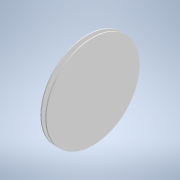
# Autodesk Inventor part: Base Plate
Saved by Autodesk Inventor 2021 (Build 250183000, 183)
## iProperties
Created: 2021-05-31
Part Number: Base Plate
Material: Generic
Document SubType Name: Modeling
Designer: techv
Density: 1 g/cm^3
Appearance: Default
Author: techv
Autodesk Inventor part; units mm, degrees
ref_plane "YZ Plane" through (0, 0, 0) normal (1, 0, 0) x (0, 1, 0)
ref_plane "XZ Plane" through (0, 0, 0) normal (0, 1, 0) x (-1, 0, 0)
ref_plane "XY Plane" through (0, 0, 0) normal (0, 0, 1) x (1, 0, 0)
sketch "Sketch1" plane through (0, 0, 0) normal (1, 0, 0) x (0, 1, 0)
  circle A0 centre (0, 0) radius 125
  dimension "d0" = 250
  constraints: 1 centre point, 1 coincident
  measures "d0" diameter of A0
extrude "Extrusion1" add sketch "Sketch1" along normal blind 3
sketch "Sketch2" plane through (3, 0, 0) normal (1, 0, 0) x (0, 0, -1)
  circle A0 centre (0, 0) radius 15
  line L0 (0, 0) -> (0, 70) construction
  circle A1 centre (0, 70) radius 7.5
  circle A2 centre (-49.4975, 49.4975) radius 7.5
  circle A3 centre (-70, 0) radius 7.5
  circle A4 centre (-49.4975, -49.4975) radius 7.5
  circle A5 centre (0, -70) radius 7.5
  circle A6 centre (49.4975, -49.4975) radius 7.5
  circle A7 centre (70, 0) radius 7.5
  circle A8 centre (49.4975, 49.4975) radius 7.5
  line L1 (0, 0) -> (92.388, 38.2683) construction
  line L2 (0, 0) -> (100, 0) construction
  circle A9 centre (92.388, 38.2683) radius 7.5
  circle A10 centre (38.2683, 92.388) radius 7.5
  circle A11 centre (-38.2683, 92.388) radius 7.5
  circle A12 centre (-92.388, 38.2683) radius 7.5
  circle A13 centre (-92.388, -38.2683) radius 7.5
  circle A14 centre (-38.2683, -92.388) radius 7.5
  circle A15 centre (38.2683, -92.388) radius 7.5
  circle A16 centre (92.388, -38.2683) radius 7.5
  dimension "d3" = 30
  dimension "d4" = 70
  dimension "d5" = 15
  dimension "d8" = 360
  dimension "d10" = 100
  dimension "d11" = 22.5
  dimension "d12" = 15
  dimension "d15" = 360
  constraints: 17 centre point, 6 end point, 3 coincident, 1 equal length, 1 horizontal, 1 vertical, 34 other
  measures "d3" diameter of A0
  measures "d4" distance of L0.start L0.end
  measures "d5" diameter of A1
  measures "d10" distance of L0.start L1.end
  measures "d11" angle of L2 L1
  measures "d12" diameter of A9
extrude "Extrusion2" add sketch "Sketch2" along normal blind 10 contours A1 | A2 | A3 | A4 | A5 | A6 | A7 | A8 | A9 | A10 | A11 | A12 | A13 | A14 | A15 | A16
ref_plane "Work Plane1" through (8, -49.4975, 49.4975) normal (1, 0, 0) x (0, 0, -1)
mirror "Mirror1" about plane through (8, -49.4975, 49.4975) normal (1, 0, 0) of "Extrusion1"
sketch "Sketch3" plane through (16, 0, 0) normal (1, 0, 0) x (0, 0, -1)
  circle A0 centre (0, 0) radius 15
  dimension "d20" = 30
  constraints: 1 centre point, 1 coincident
  measures "d20" diameter of A0
extrude "Extrusion3" cut sketch "Sketch3" against normal through all
body "Solid1"
